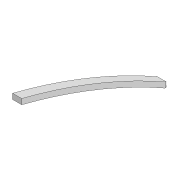
# Autodesk Inventor part: Part_8_p1
Saved by Autodesk Inventor 2022 (Build 260153000, 153)
## iProperties
Created: 2022-04-24
Part Number: Part_8_p1
Material: Generic
Document SubType Name: Modeling
Designer: dell
Density: 1 g/cm^3
Appearance: Default
Author: dell
Autodesk Inventor part; units mm, degrees
ref_plane "YZ Plane" through (0, 0, 0) normal (1, 0, 0) x (0, 1, 0)
ref_plane "XZ Plane" through (0, 0, 0) normal (0, 1, 0) x (-1, 0, 0)
ref_plane "XY Plane" through (0, 0, 0) normal (0, 0, 1) x (1, 0, 0)
sketch "Sketch1" plane through (0, 0, 0) normal (0, 1, 0) x (-1, 0, 0)
  line L0 (0, 0) -> (0, -180) construction
  line L1 (5, 0) -> (5, -180)
  line L2 (-5, -180) -> (-5, 0)
  arc A0 (5, 0) -> (-5, 0) centre (0, 0) ccw
  arc A1 (-5, -180) -> (5, -180) centre (0, -180) ccw
  circle A2 centre (0, 0) radius 1.65
  line L3 (0, -40) -> (0, -140) construction
  line L4 (1.65, -40) -> (1.65, -140)
  line L5 (-1.65, -140) -> (-1.65, -40)
  arc A3 (1.65, -40) -> (-1.65, -40) centre (0, -40) ccw
  arc A4 (-1.65, -140) -> (1.65, -140) centre (0, -140) ccw
  point P0 (0, -90)
  point P1 (0, -90)
  dimension "d0" = 180
  dimension "d1" = 10
  dimension "d2" = 3.3
  dimension "d3" = 40
  dimension "d5" = 140
  dimension "d6" = 3.3
  constraints: 16 end point, 8 point on circle, 8 tangent, 5 centre point, 2 midpoint, 2 parallel, 2 point on line, 1 coincident, 1 vertical
  measures "d0" distance of L0.end L0.start
  measures "d1" distance between parallel lines of L1 L2
  measures "d2" diameter of A2
  measures "d3" distance of L0.start L3.start
  measures "d5" distance of L0.start L3.end
  measures "d6" distance between parallel lines of L5 L4
extrude "Extrusion1" add sketch "Sketch1" along normal blind 6
sketch "Sketch2" plane through (5, 0, 0) normal (1, 0, 0) x (0, 0, -1)
  line L0 (180, 0) -> (180, 6) projected
  line L1 (0, 0) -> (180, 0) projected
  line L2 (180, 0) -> (180, 6) projected
  line L3 (0, 6) -> (180, 6) projected
  line L4 (0, 0) -> (0, 6) projected
  line L5 (180, 0) -> (180, 0) projected
  line L6 (180, 0) -> (180, 6) projected
  line L7 (180, 6) -> (180, 6) projected
  line L8 (180, 0) -> (180, 6) projected
  line L9 (180, 0) -> (0, 0) projected
  arc A0 (498.004, -84) -> (180, 0) centre (180, -643.9437) ccw
  line L10 (180, 6) -> (0, 6) projected
  arc A1 (498.004, -78) -> (180, 6) centre (180, -637.9437) ccw
  line L11 (498.004, -78) -> (498.004, -84)
  line L12 (0, 0) -> (180, 0) projected
  dimension "d9" = 6
  dimension "d10" = 498.004
  dimension "d11" = 90
  constraints: 4 point on circle, 2 centre point, 2 end point, 2 tangent, 1 vertical
  measures "d9" distance of L11.start L11.end
  measures "d10" distance between parallel lines of L4 L11
  measures "d11" distance from line of L3 L11.end
extrude "Extrusion2" add sketch "Sketch2" against normal blind 10 contours L0 A1 L11 A0
fillet "Fillet1" radius 2 4 edges at (0, -78, -498.004) (5, -81, -498.004) (-5, -81, -498.004) (0, -84, -498.004)
sketch "Sketch3" plane through (0, 6, 0) normal (0, 1, 0) x (1, 0, 0)
  line L0 (-25.1236, -17.4365) -> (19.1239, -17.4365)
  line L1 (19.1239, -17.4365) -> (19.1239, 173.8027)
  line L2 (19.1239, 173.8027) -> (-25.1236, 173.8027)
  line L3 (-25.1236, 173.8027) -> (-25.1236, -17.4365)
  line L4 (-48.0471, -35.7333) -> (42.457, -35.7333)
  line L5 (42.457, -35.7333) -> (42.457, 337.7497)
  line L6 (42.457, 337.7497) -> (-48.0471, 337.7497)
  line L7 (-48.0471, 337.7497) -> (-48.0471, -35.7333)
  line L8 (-102.0639, -92.3443) -> (98.6132, -92.3443)
  line L9 (98.6132, -92.3443) -> (98.6132, 617.9416)
  line L10 (98.6132, 617.9416) -> (-102.0639, 617.9416)
  line L11 (-102.0639, 617.9416) -> (-102.0639, -92.3443)
  point P0 (0, 0)
  constraints: 24 end point, 6 parallel, 3 horizontal, 3 perpendicular
extrude "Extrusion3" cut sketch "Sketch3" against normal blind 100 contours L3 L2 L1 L0 | L7 L6 L5 L4
body "Solid1"
